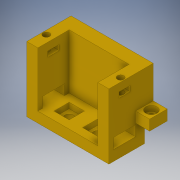
# Autodesk Inventor part: HIP
Saved by Autodesk Inventor 2017 (Build 210142000, 142)
## iProperties
Created: 2018-07-28
Part Number: HIP
Material: Generic
Document SubType Name: Modeling
Designer: Alexander Miller
Density: 1 g/cm^3
Appearance: Gold
Author: Alexander Miller
Autodesk Inventor part; units mm, degrees
ref_plane "YZ Plane" through (0, 0, 0) normal (1, 0, 0) x (0, 1, 0)
ref_plane "XZ Plane" through (0, 0, 0) normal (0, 1, 0) x (-1, 0, 0)
ref_plane "XY Plane" through (0, 0, 0) normal (0, 0, 1) x (1, 0, 0)
sketch "Sketch1" plane through (0, 0, 0) normal (0, 0, 1) x (1, 0, 0)
  line L0 (-15.75, 17) -> (15.75, 17)
  line L1 (15.75, 17) -> (15.75, -17)
  line L2 (15.75, -17) -> (-15.75, -17)
  line L3 (-15.75, -17) -> (-15.75, 17)
  point P0 (0, 0)
  point P1 (15.75, 0)
  point P2 (0, 17)
  dimension "d0" = 34
  dimension "d1" = 31.5
  constraints: 8 end point, 2 midpoint, 2 parallel, 1 horizontal, 1 horizontal alignment, 1 perpendicular, 1 vertical alignment
  measures "d0" distance of L0.end L1.end
  measures "d1" distance of L0.start L0.end
extrude "Extrusion1" add sketch "Sketch1" along normal blind 2
sketch "Sketch2" plane through (0, 0, 2) normal (0, 0, 1) x (1, 0, 0)
  line L0 (-11.5, 8) -> (-15.75, 8)
  line L1 (-15.75, 8) -> (-15.75, -13)
  line L2 (-15.75, -13) -> (-11.5, -13)
  line L3 (-11.5, -13) -> (-11.5, 8)
  line L4 (11.5, 8) -> (15.75, 8)
  line L5 (15.75, 8) -> (15.75, -13)
  line L6 (15.75, -13) -> (11.5, -13)
  line L7 (11.5, -13) -> (11.5, 8)
  line L8 (15.75, -13) -> (-15.75, -13)
  line L9 (-15.75, -13) -> (-15.75, -17)
  line L10 (-15.75, -17) -> (15.75, -17)
  line L11 (15.75, -17) -> (15.75, -13)
  line L12 (-15.75, 17) -> (-15.75, -17) projected
  line L13 (15.75, 17) -> (-15.75, 17) projected
  line L14 (15.75, -17) -> (15.75, 17) projected
  line L15 (-15.75, -17) -> (15.75, -17) projected
  point P0 (0, 0)
  dimension "d4" = 23
  dimension "d5" = 4
  dimension "d67" = 21
  constraints: 24 end point, 8 collinear, 6 parallel, 3 horizontal, 3 perpendicular, 1 point on line
  measures "d4" distance between parallel lines of L7 L3
  measures "d5" distance between parallel lines of L10 L8
  measures "d67" distance between parallel lines of L2 L0
extrude "Extrusion2" add sketch "Sketch2" along normal blind 12 contours L3 L2 L1 L0 | L8 L6 L11 L10 L9 L2 | L7 L4 L5 L6
sketch "Sketch8" plane through (-11.5, -13, 2) normal (0, 1, 0) x (1, 0, 0)
  circle A0 centre (6, -6) radius 6 construction
  circle A1 centre (17, -6) radius 6 construction
  line L0 (0, 0) -> (0, -12) construction
  line L1 (23, -12) -> (0, -12) construction
  line L2 (0, 0) -> (23, 0) construction
  line L3 (23, 0) -> (23, -12) construction
  circle A2 centre (6, -6) radius 1.675
  circle A3 centre (17, -6) radius 1.675
  point P0 (11.5, 2)
  dimension "d29" = 3.35
  constraints: 6 tangent, 4 centre point, 2 coincident, 1 equal radius
  measures "d29" diameter of A2
extrude "Extrusion8" cut sketch "Sketch8" against normal through all
sketch "Sketch9" plane through (-11.5, -13, 2) normal (0, 1, 0) x (1, 0, 0)
  line L0 (3.075, -8.925) -> (8.925, -8.925)
  line L1 (8.925, -8.925) -> (8.925, -3.075)
  line L2 (8.925, -3.075) -> (3.075, -3.075)
  line L3 (3.075, -3.075) -> (3.075, -8.925)
  line L4 (14.075, -8.925) -> (19.925, -8.925)
  line L5 (19.925, -8.925) -> (19.925, -3.075)
  line L6 (19.925, -3.075) -> (14.075, -3.075)
  line L7 (14.075, -3.075) -> (14.075, -8.925)
  circle A0 centre (6, -6) radius 1.675 projected
  circle A1 centre (17, -6) radius 1.675 projected
  point P0 (11.5, 2)
  point P1 (6, -3.075)
  point P2 (17, -3.075)
  point P3 (3.075, -6)
  point P4 (14.075, -6)
  dimension "d32" = 5.85
  constraints: 16 end point, 4 midpoint, 4 parallel, 2 equal length, 2 horizontal, 2 horizontal alignment, 2 perpendicular, 2 vertical alignment, 1 point on line
  measures "d32" distance of L1.end L2.end
extrude "Extrusion9" cut sketch "Sketch9" against normal blind 2.15
sketch "Sketch10" plane through (0, 0, 0) normal (0, 0, -1) x (-1, 0, 0)
  line L0 (-15.75, 17) -> (15.75, 17)
  line L1 (15.75, 17) -> (15.75, -12)
  line L2 (15.75, -12) -> (-15.75, -12)
  line L3 (-15.75, -12) -> (-15.75, 17)
  line L4 (-15.75, -17) -> (15.75, -17) projected
  line L5 (15.75, 17) -> (-15.75, 17) projected
  line L6 (-15.75, 17) -> (-15.75, -17) projected
  point P0 (0, 0)
  point P1 (0, 17)
  point P2 (15.75, 2.5)
  dimension "d36" = 29
  constraints: 8 end point, 2 collinear, 2 midpoint, 2 parallel, 1 horizontal, 1 perpendicular, 1 vertical alignment
  measures "d36" distance of L2.end L0.start
extrude "Extrusion10" add sketch "Sketch10" along normal blind 3
sketch "Sketch16" plane through (15.75, -17, 14) normal (1, 0, 0) x (0, 0, -1)
  line L0 (1.75, 8) -> (10.25, 8)
  line L1 (10.25, 8) -> (10.25, 4)
  line L2 (10.25, 4) -> (1.75, 4)
  line L3 (1.75, 4) -> (1.75, 8)
  line L4 (12, 4) -> (0, 4) projected
  point P0 (14, 17)
  point P1 (6, 8)
  point P2 (6, 4)
  point P3 (6, 4)
  dimension "d62" = 8.5
  dimension "d63" = 4
  constraints: 8 end point, 3 midpoint, 2 parallel, 2 vertical alignment, 1 collinear, 1 horizontal, 1 perpendicular
  measures "d62" distance of L0.start L0.end
  measures "d63" distance of L0.end L1.end
extrude "Extrusion16" cut sketch "Sketch16" against normal through all
sketch "Sketch20" plane through (-15.75, 8, 2) normal (0, 1, 0) x (1, 0, 0)
  circle A0 centre (1.5, -6) radius 1.25
  circle A1 centre (30, -6) radius 1.25
  line L0 (4.25, -12) -> (0, -12) projected
  line L1 (4.25, 0) -> (4.25, -12) projected
  line L2 (27.25, 0) -> (27.25, -12) projected
  point P0 (15.75, 2)
  point P1 (4.25, -6)
  dimension "d90" = 2.5
  dimension "d92" = 1.5
  dimension "d93" = 1.5
  constraints: 2 centre point, 2 horizontal alignment, 1 equal radius, 1 midpoint
  measures "d90" diameter of A0
  measures "d92" distance edge to line of A0 L1
  measures "d93" distance edge to line of A1 L2
extrude "Extrusion20" cut sketch "Sketch20" against normal blind 10
sketch "Sketch21" plane through (-15.75, -17, 14) normal (-1, 0, 0) x (0, 0, 1)
  line L0 (-17, 12.5) -> (-10.25, 12.5)
  line L1 (-10.25, 12.5) -> (-10.25, 8.5)
  line L2 (-10.25, 8.5) -> (-17, 8.5)
  line L3 (-17, 8.5) -> (-17, 12.5)
  line L4 (-14, 0) -> (0, 0) projected
  line L5 (-17, 5) -> (-17, 34) projected
  point P0 (-14, 17)
  point P1 (-17, 7)
  point P2 (-10.25, 8)
  dimension "d96" = 8.5
  dimension "d100" = 4
  constraints: 8 end point, 2 parallel, 1 collinear, 1 horizontal, 1 perpendicular, 1 vertical alignment
  measures "d96" distance between parallel lines of L4 L2
  measures "d100" distance of L2.end L0.start
extrude "Extrusion21" add sketch "Sketch21" along normal blind 5.35
sketch "Sketch24" plane through (15.75, -17, 14) normal (1, 0, 0) x (0, 0, -1)
  line L0 (10.25, 12.5) -> (17, 12.5)
  line L1 (17, 12.5) -> (17, 8.5)
  line L2 (17, 8.5) -> (10.25, 8.5)
  line L3 (10.25, 8.5) -> (10.25, 12.5)
  line L4 (17, 34) -> (17, 5) projected
  line L5 (14, 0) -> (0, 0) projected
  point P0 (14, 17)
  point P1 (17, 7)
  point P2 (10.25, 8)
  dimension "d107" = 8.5
  dimension "d108" = 4
  constraints: 8 end point, 2 parallel, 1 collinear, 1 horizontal, 1 perpendicular, 1 vertical alignment
  measures "d107" distance between parallel lines of L5 L2
  measures "d108" distance of L2.end L0.start
extrude "Extrusion24" add sketch "Sketch24" along normal blind 5.35
sketch "Sketch22" plane through (-15.75, -4.5, 3.75) normal (0, 1, 0) x (1, 0, 0)
  circle A0 centre (-2.675, 3.375) radius 1.175
  line L0 (-5.35, 0) -> (-5.35, 6.75) projected
  line L1 (0, 0) -> (-5.35, 0) projected
  circle A1 centre (34.175, 3.375) radius 1.175
  line L2 (31.5, 0) -> (36.85, 0) projected
  point P0 (15.75, 3.75)
  point P1 (-5.35, 3.375)
  point P2 (-2.675, 0)
  point P3 (34.175, 0)
  dimension "d101" = 2.35
  constraints: 3 midpoint, 2 centre point, 2 horizontal alignment, 2 vertical alignment, 1 equal radius
  measures "d101" diameter of A0
extrude "Extrusion22" cut sketch "Sketch22" against normal through all
sketch "Sketch23" plane through (-15.75, -4.5, 3.75) normal (0, 1, 0) x (1, 0, 0)
  circle A0 centre (-2.675, 3.375) radius 2.175
  circle A1 centre (-2.675, 3.375) radius 1.175 projected
  circle A2 centre (34.175, 3.375) radius 2.175
  circle A3 centre (34.175, 3.375) radius 1.175 projected
  point P0 (15.75, 3.75)
  dimension "d104" = 4.35
  constraints: 2 centre point, 2 concentric, 1 equal radius
  measures "d104" diameter of A0
extrude "Extrusion23" cut sketch "Sketch23" against normal blind 2
sketch "Sketch25" plane through (15.75, -17, 14) normal (1, 0, 0) x (0, 0, -1)
  line L0 (3.825, 22.075) -> (8.175, 22.075)
  line L1 (8.175, 22.075) -> (8.175, 20)
  line L2 (8.175, 20) -> (3.825, 20)
  line L3 (3.825, 20) -> (3.825, 22.075)
  line L4 (12, 25) -> (0, 25) projected
  point P0 (14, 17)
  point P1 (6, 25)
  point P2 (6, 22.075)
  dimension "d111" = 5
  dimension "d112" = 2.075
  dimension "d113" = 4.35
  constraints: 8 end point, 2 midpoint, 2 parallel, 1 horizontal, 1 perpendicular, 1 vertical alignment
  measures "d111" distance between parallel lines of L2 L4
  measures "d112" distance of L2.end L0.start
  measures "d113" distance of L1.end L2.end
extrude "Extrusion25" cut sketch "Sketch25" against normal through all
sketch "Sketch26" plane through (0, 0, 2) normal (0, 0, 1) x (1, 0, 0)
  line L0 (-15.75, 17) -> (15.75, 17)
  line L1 (15.75, 17) -> (15.75, 8)
  line L2 (15.75, 8) -> (-15.75, 8)
  line L3 (-15.75, 8) -> (-15.75, 17)
  line L4 (11.5, 8) -> (15.75, 8) projected
  line L5 (15.75, 8) -> (15.75, 17) projected
  line L6 (-15.75, 17) -> (-15.75, 8) projected
  line L7 (15.75, 17) -> (-15.75, 17) projected
  point P0 (0, 0)
  constraints: 8 end point, 4 collinear, 2 parallel, 1 horizontal, 1 perpendicular
extrude "Extrusion26" cut sketch "Sketch26" against normal through all
sketch "Sketch27" plane through (0, 0, 0) normal (0, 0, -1) x (-1, 0, 0)
  line L0 (-15.75, -17) -> (15.75, -17) projected
  line L1 (15.75, -12) -> (-15.75, -12) projected
  line L2 (15.75, -17) -> (-15.75, -17)
  line L3 (-15.75, -17) -> (-15.75, -12)
  line L4 (-15.75, -12) -> (15.75, -12)
  line L5 (15.75, -12) -> (15.75, -17)
  point P0 (0, 0)
  constraints: 8 end point, 2 parallel, 1 horizontal, 1 perpendicular
extrude "Extrusion27" cut sketch "Sketch27" against normal blind 0.3
equation "\"d1\" = servo_D"
equation "\"d4\" = servo_A"
equation "\"d5\" = bot_mat"
equation "\"d67\" = servo_E"
equation "\"d6\" = servo_B"
equation "\"d33\" = nut_B"
equation "\"d92\" = servo_L"
equation "\"d93\" = d92"
equation "\"d109\" = d97"
equation "\"d112\" = nut_B_1 + Tolerance"
equation "\"d113\" = nut_A_1"
equation "\"bot_mat\" = 4"
equation "\"servo_D\" = 31.5"
equation "\"servo_A\" = 23"
equation "\"servo_E\" = 21"
equation "\"servo_B\" = 12"
equation "\"nut_B\" = 2.15"
equation "\"servo_L\" = 1.5"
equation "\"d97\" = 5.35"
equation "\"nut_B_1\" = 1.725"
equation "\"Tolerance\" = 0.35"
equation "\"nut_A_1\" = 4.35"
body "Solid1"
